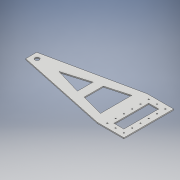
# Autodesk Inventor part: W1support
Saved by Autodesk Inventor 2017 (Build 210142000, 142)
## iProperties
Created: 2016-10-18
Part Number: W1support
Material: Generic
Document SubType Name: Sheet Metal
Designer: aesen
Density: 1 g/cm^3
Sheet Metal Rule: Default_mm
Appearance: Default
Author: aesen
Autodesk Inventor part; units mm, degrees
ref_plane "YZ Plane" through (0, 0, 0) normal (1, 0, 0) x (0, 1, 0)
ref_plane "XZ Plane" through (0, 0, 0) normal (0, 1, 0) x (-1, 0, 0)
ref_plane "XY Plane" through (0, 0, 0) normal (0, 0, 1) x (1, 0, 0)
sketch "Sketch1" plane through (0, 0, 0) normal (0, 0, 1) x (1, 0, 0)
  line L0 (83.0359, 109.6863) -> (83.0359, -6.9318)
  line L1 (255.4191, -98.6226) -> (-294.5809, 18.2835)
  line L2 (-294.5809, 84.4713) -> (-294.5809, 18.2835)
  line L3 (255.4191, 201.3774) -> (-294.5809, 84.4713)
  line L4 (-126.7462, 51.3687) -> (31.6101, 98.6927)
  line L5 (31.6102, 4.0618) -> (-126.7462, 51.3687)
  line L6 (31.6102, 4.0618) -> (31.6101, 98.6927)
  line L7 (415.4191, -98.6226) -> (415.4191, 201.3774)
  line L8 (370.1461, -53.6226) -> (370.1461, 156.3774)
  line L9 (310.1461, 156.3774) -> (310.1461, -53.6226)
  circle A0 centre (290.1461, 76.3774) radius 3.5
  circle A1 centre (290.1461, 26.3774) radius 3.5
  circle A2 centre (390.1461, -23.6226) radius 3.5
  circle A3 centre (290.1461, -23.6226) radius 3.5
  circle A4 centre (390.1461, -73.6226) radius 3.5
  line L10 (217.7103, -43.1749) -> (217.7103, 145.9755)
  line L11 (83.0359, -6.9318) -> (218.5191, -43.3926)
  line L12 (83.0359, 109.6863) -> (217.7103, 145.9755)
  line L13 (255.4191, -98.6226) -> (415.4191, -98.6226)
  line L14 (310.1461, -53.6226) -> (370.1461, -53.6226)
  circle A5 centre (290.1461, -73.6226) radius 3.7075
  circle A6 centre (340.1461, -73.6226) radius 3.5
  circle A7 centre (390.3597, 26.3774) radius 3.5
  circle A8 centre (390.1461, 76.3774) radius 3.5
  circle A9 centre (290.1461, 126.3774) radius 3.5
  circle A10 centre (390.1461, 126.3774) radius 3.5
  circle A11 centre (340.1461, 176.3774) radius 3.5
  line L15 (370.1461, 156.3774) -> (310.1461, 156.3774)
  circle A12 centre (390.1461, 176.3774) radius 3.7075
  line L16 (415.4191, 201.3774) -> (255.4191, 201.3774)
  circle A13 centre (290.1461, 176.3774) radius 3.5
  circle A14 centre (-258.8694, 51.3773) radius 12.7
  point P0 (0, 0)
  point P1 (0, 0)
  dimension "d4" = 25.4
  dimension "d5" = 39.7957
  dimension "d6" = 39.7954
  constraints: 34 end point, 15 centre point, 1 point on line
  measures "d4" diameter of A14
  measures "d5" distance from line of L3 A14.centre
  measures "d6" distance from line of L1 A14.centre
extrude "Extrusion2" add sketch "Sketch1" along normal blind 6.35
equation "\"BendRadius\" = Thickness"
equation "\"BendReliefWidth\" = Thickness"
equation "\"BendReliefDepth\" = 0.5 * Thickness"
equation "\"CornerReliefSize\" = 4 * Thickness"
equation "\"MinimumRemnant\" = 2 * Thickness"
equation "\"TransitionRadius\" = BendRadius"
equation "\"JacobiRadiusSize\" = BendRadius"
equation "\"GapSize\" = Thickness"
equation "\"Thickness\" = 0.5"
body "Solid2"
